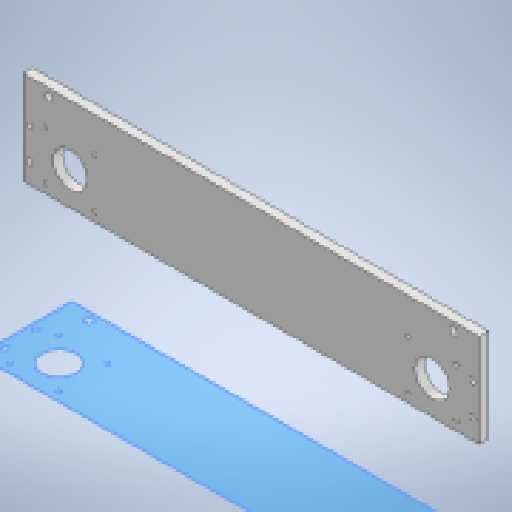
# Autodesk Inventor part: креп_мотора
Saved by Autodesk Inventor 2023.1 (Build 271208000, 208)
## iProperties
Created: 2025-12-22
Part Number: креп_мотора
Material: Типовые
Document SubType Name: Modeling
Designer: DELL
Density: 1 g/cm^3
Appearance: По умолчанию
Author: DELL
Autodesk Inventor part; units mm, degrees
ref_plane "YZ Plane" through (0, 0, 0) normal (1, 0, 0) x (0, 1, 0)
ref_plane "XZ Plane" through (0, 0, 0) normal (0, 1, 0) x (-1, 0, 0)
ref_plane "XY Plane" through (0, 0, 0) normal (0, 0, 1) x (1, 0, 0)
sketch "Эскиз1" plane through (0, 0, 0) normal (0, 0, 1) x (1, 0, 0)
  line L0 (-26.0621, -17.2379) -> (-22.2379, -21.0621) construction
  arc A0 (-22.2379, -21.0621) -> (-22.0257, -21.15) centre (-22.0257, -20.85) ccw construction
  line L1 (-22.0257, -21.15) -> (12.0257, -21.15) construction
  arc A1 (12.0257, -21.15) -> (12.2379, -21.0621) centre (12.0257, -20.85) ccw construction
  line L2 (12.2379, -21.0621) -> (16.0621, -17.2379) construction
  arc A2 (16.0621, -17.2379) -> (16.15, -17.0257) centre (15.85, -17.0257) ccw construction
  line L3 (16.15, -17.0257) -> (16.15, 17.0257) construction
  arc A3 (16.15, 17.0257) -> (16.0621, 17.2379) centre (15.85, 17.0257) ccw construction
  line L4 (16.0621, 17.2379) -> (12.2379, 21.0621) construction
  arc A4 (12.2379, 21.0621) -> (12.0257, 21.15) centre (12.0257, 20.85) ccw construction
  line L5 (12.0257, 21.15) -> (-22.0257, 21.15) construction
  arc A5 (-22.0257, 21.15) -> (-22.2379, 21.0621) centre (-22.0257, 20.85) ccw construction
  line L6 (-22.2379, 21.0621) -> (-26.0621, 17.2379) construction
  arc A6 (-26.0621, 17.2379) -> (-26.15, 17.0257) centre (-25.85, 17.0257) ccw construction
  line L7 (-26.15, 17.0257) -> (-26.15, -17.0257) construction
  arc A7 (-26.15, -17.0257) -> (-26.0621, -17.2379) centre (-25.85, -17.0257) ccw construction
  circle A8 centre (-5, 0) radius 11 projected
  circle A9 centre (-20.5, 15.5) radius 1.25 projected
  circle A10 centre (10.5, 15.5) radius 1.25 projected
  circle A11 centre (10.5, -15.5) radius 1.25 projected
  circle A12 centre (-20.5, -15.5) radius 1.25 projected
  circle A13 centre (20.65, -8.65) radius 1.75 projected
  circle A14 centre (20.65, 11.35) radius 1.75 projected
  line L8 (-255.65, -21.15) -> (25.15, -21.15)
  line L9 (25.15, -21.15) -> (25.15, 38.85)
  line L10 (25.15, 38.85) -> (-255.65, 38.85)
  line L11 (-255.65, 38.85) -> (-255.65, -21.15)
  line L12 (-255.65, -21.15) -> (25.15, 38.85) construction
  line L13 (25.15, -21.15) -> (-255.65, 38.85) construction
  line L14 (-115.25, 8.85) -> (-115.25, -21.15) construction
  circle A15 centre (-210, 15.5) radius 1.25
  circle A16 centre (-241, 15.5) radius 1.25
  circle A17 centre (-241, -15.5) radius 1.25
  circle A18 centre (-210, -15.5) radius 1.25
  circle A19 centre (-251.15, -8.65) radius 1.75
  circle A20 centre (-251.15, 11.35) radius 1.75
  circle A21 centre (-225.5, 0) radius 11
  circle A22 centre (8.65, 58.4393) radius 2.1 projected
  circle A23 centre (-244.15, 33.15) radius 2.5 projected
  circle A24 centre (13.65, 33.15) radius 2.5 projected
  point P0 (-5, -21.15)
  dimension "d8" = 280.8
  dimension "d9" = 60
  dimension "d10" = 4.5
  constraints: 14 end point, 7 centre point, 7 symmetric about line, 4 midpoint, 2 parallel, 1 horizontal, 1 perpendicular, 1 point on line, 7 other
  measures "d8" distance of L10.end L9.end
  measures "d9" distance of L8.end L9.end
  measures "d10" distance from line of L9 A13.centre
extrude "Выдавливание1" add sketch "Эскиз1" along normal blind 6 contours L11 L10 L9 L8
